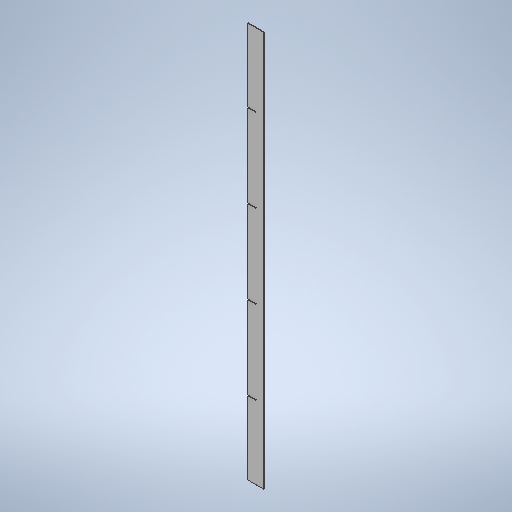
# Autodesk Inventor part: BSH 046 stringer 6
Saved by Autodesk Inventor 2025 (Build 290162010, 162A)
## iProperties
Created: 2024-07-23
Part Number: BSH 046 stringer 6
Material: 09g2s
Document SubType Name: Sheet Metal
Designer: admin
Density: 7.85 g/cm^3
Sheet Metal Rule: AISI304 3mm Die 32
Sheet Metal Width: 95,000 mm
Sheet Metal Length: 2380,000 mm
Sheet Metal Area: 226100,000 mm^2
Appearance: Default
Mass: 5310.04 g
Surface Area: 4669.72 cm^2
Volume: 676.438 cm^3
Flat Pattern Width: 9.5 cm
Flat Pattern Length: 238 cm
Flat Pattern Area: 2261 cm^2
Author: admin
Autodesk Inventor part; units mm, degrees
ref_plane "YZ Plane" through (0, 0, 0) normal (1, 0, 0) x (0, 1, 0)
ref_plane "XZ Plane" through (0, 0, 0) normal (0, 1, 0) x (-1, 0, 0)
ref_plane "XY Plane" through (0, 0, 0) normal (0, 0, 1) x (1, 0, 0)
sketch "Sketch6" plane through (0, 0, 0) normal (0, 1, 0) x (-1, 0, 0)
  line L0 (0, -1190) -> (-95, -1190)
  line L1 (-95, -1190) -> (-95, 1190)
  line L2 (-95, 1190) -> (0, 1190)
  line L3 (0, 1190) -> (0, -1190)
  point P0 (-4059.1747, 1994.2978)
  point P1 (0, 0)
  point P2 (0, 0)
  dimension "d26" = 95
  dimension "d27" = 2380
  measures "d26" distance of L1.end L2.end
  measures "d27" distance of L0.end L1.end
extrude "Plate4" add sketch "Sketch6" along normal blind 3
sketch "Sketch7" plane through (0, 0, 0) normal (0, -1, 0) x (1, 0, 0)
  line L0 (0, 1190) -> (95, 1190) projected
  line L1 (0, -1190) -> (0, 1190) projected
  line L2 (95, -1190) -> (0, -1190) projected
  line L3 (95, 1190) -> (95, -1190) projected
  line L4 (0, -747.363) -> (48.5, -747.363)
  line L5 (48.5, -747.363) -> (48.5, -750.563)
  line L6 (48.5, -750.563) -> (0, -750.563)
  line L7 (0, -750.563) -> (0, -747.363)
  point P0 (0, 0)
  point P1 (0, -750.563)
  point P2 (0, 200)
  point P3 (46.4173, 200)
  point P4 (0, -750.563)
  dimension "d29" = 48.5
  dimension "d30" = 3.2
  dimension "d31" = 439.437
  constraints: 8 end point, 2 parallel, 1 horizontal, 1 perpendicular, 1 point on line
  measures "d29" distance of L5.end L6.end
  measures "d30" distance of L4.end L5.end
  measures "d31" distance between parallel lines of L2 L6
extrude "Extrusion2" cut sketch "Sketch7" against normal through all contours L4 L5 L6 L1
pattern_linear "Rectangular Pattern1" count 5 spacing 500 along (0, 0, 1) of "Extrusion2"
equation "\"d28\" = Thickness"
equation "\"BendReliefWidth\" = Thickness"
equation "\"BendReliefDepth\" = 0.5 * Thickness"
equation "\"CornerReliefSize\" = 4 * Thickness"
equation "\"MinimumRemnant\" = 2 * Thickness"
equation "\"TransitionRadius\" = BendRadius"
equation "\"JacobiRadiusSize\" = BendRadius"
equation "\"GapSize\" = Thickness"
equation "\"Thickness\" = 3"
equation "\"BendRadius\" = 5"
body "Solid2"
